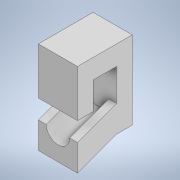
# Autodesk Inventor part: top_part
Saved by Autodesk Inventor 2021 (Build 250183000, 183)
## iProperties
Created: 2021-04-02
Part Number: top_part
Material: Generic
Document SubType Name: Modeling
Designer: Jawal
Density: 1 g/cm^3
Appearance: Default
Author: Jawal
Autodesk Inventor part; units mm, degrees
ref_plane "YZ Plane" through (0, 0, 0) normal (1, 0, 0) x (0, 1, 0)
ref_plane "XZ Plane" through (0, 0, 0) normal (0, 1, 0) x (-1, 0, 0)
sketch "Sketch1" plane through (0, 0, 0) normal (0, 0, 1) x (1, 0, 0)
  line L0 (-12.5, 12.5) -> (12.5, 12.5)
  line L1 (12.5, 12.5) -> (12.5, -37.5)
  line L2 (12.5, -37.5) -> (-12.5, -37.5)
  line L3 (-12.5, -37.5) -> (-12.5, 12.5)
  point P0 (0, 0)
  dimension "d0" = 25
  dimension "d1" = 50
  dimension "d2" = 12.5
  dimension "d3" = 12.5
  constraints: 8 end point, 2 parallel, 1 horizontal, 1 perpendicular
  measures "d0" distance of L0.start L0.end
  measures "d1" distance of L0.end L1.end
  measures "d2" distance from line of L1 point (0, 0)
  measures "d3" distance from line of point (0, 0) L0
extrude "Extrusion1" add sketch "Sketch1" along normal blind 10
sketch "Sketch2" plane through (0, 0, 0) normal (0, 0, -1) x (-1, 0, 0)
  circle A0 centre (0, -33) radius 1.5
  circle A1 centre (0, 0) radius 7.5
  dimension "d7" = 3
  dimension "d8" = 33
  dimension "d17" = 15
  constraints: 2 centre point, 1 coincident
  measures "d7" diameter of A0
  measures "d8" distance of A0.centre point (0, 0)
  measures "d17" diameter of A1
extrude "Extrusion2" add sketch "Sketch2" along normal blind 6 contours A0
sketch "Sketch3" plane through (0, 0, 10) normal (0, 0, 1) x (1, 0, 0)
  arc A0 (7.5, 0) -> (-7.5, 0) centre (0, 0) ccw
  line L0 (-7.5, 0) -> (-12.5, 0)
  line L1 (-12.5, 12.5) -> (-12.5, -37.5) projected
  line L2 (-12.5, 0) -> (-12.5, 12.5)
  line L3 (12.5, 12.5) -> (-12.5, 12.5) projected
  line L4 (12.5, 12.5) -> (12.5, 0)
  line L5 (12.5, -37.5) -> (12.5, 12.5) projected
  line L6 (7.5, 0) -> (12.5, 0)
  dimension "d11" = 15
  constraints: 8 end point, 2 point on circle, 2 point on line, 1 centre point, 1 coincident, 1 collinear, 1 horizontal, 1 perpendicular
  measures "d11" diameter of A0
extrude "Extrusion3" add sketch "Sketch3" along normal blind 15
sketch "Sketch4" plane through (0, 0, 25) normal (0, 0, 1) x (1, 0, 0)
  line L0 (-12.5, 12.5) -> (-12.5, 0) projected
  line L1 (-12.5, 12.5) -> (12.5, 12.5)
  line L2 (12.5, 12.5) -> (12.5, -17.5)
  line L3 (12.5, -17.5) -> (-12.5, -17.5)
  line L4 (-12.5, -17.5) -> (-12.5, 12.5)
  point P0 (0, 0)
  dimension "d14" = 25
  dimension "d21" = 30
  constraints: 8 end point, 2 parallel, 1 horizontal, 1 perpendicular
  measures "d14" distance of L2.end L3.end
  measures "d21" distance of L1.end L2.end
extrude "Extrusion4" add sketch "Sketch4" along normal blind 10
sketch "Sketch5" plane through (0, 0, 0) normal (0, 0, -1) x (-1, 0, 0)
  circle A0 centre (0, 0) radius 7.5
  dimension "d18" = 15
  constraints: 1 centre point, 1 coincident
  measures "d18" diameter of A0
extrude "Extrusion5" cut sketch "Sketch5" against normal blind 10
sketch "Sketch6" plane through (0, 0, 10) normal (0, 0, 1) x (1, 0, 0)
  line L0 (-12.5, -20.5) -> (-12.5, -37.5)
  line L1 (-12.5, -37.5) -> (12.5, -37.5) projected
  line L2 (-12.5, -37.5) -> (12.5, -37.5)
  line L3 (12.5, -37.5) -> (12.5, -20.5)
  line L4 (12.5, -37.5) -> (12.5, 0) projected
  arc A0 (-7.5, -20.5) -> (7.5, -20.5) centre (0, -20.5) ccw
  line L5 (-12.5, -20.5) -> (-7.5, -20.5)
  line L6 (7.5, -20.5) -> (12.5, -20.5)
  line L7 (-12.5, 0) -> (-12.5, -37.5) projected
  line L8 (-12.5, -29) -> (12.5, -29)
  point P0 (0, 0)
  dimension "d22" = 15
  dimension "d23" = 17
  dimension "d24" = 17
  constraints: 12 end point, 3 point on line, 2 horizontal, 2 point on circle, 1 centre point, 1 collinear, 1 perpendicular
  measures "d22" diameter of A0
  measures "d23" distance of L1.end L3.end
  measures "d24" distance of L0.start L0.end
ref_plane "Work Plane1" through (0, -37.5, 0) normal (-1, 0, 0) x (0, 0, 1)
sketch "Sketch8" plane through (0, -37.5, 0) normal (-1, 0, 0) x (0, 0, 1)
  line L0 (10, 0) -> (10, 37.5) projected
  line L1 (10, 8.5) -> (35, -0.5993)
  line L2 (10, 8.5) -> (36.6044, 8.5) construction
  line L3 (0, 0) -> (10, 0) projected
  point P0 (0, 37.5)
  dimension "d26" = 20
  dimension "d27" = 8.5
  dimension "d32" = 25
  constraints: 4 end point, 1 equal length, 1 horizontal, 1 point on line
  measures "d26" angle of L1 L2
  measures "d27" distance between parallel lines of L3 L2
  measures "d32" distance from line of L1.end L0
sweep "Sweep1" add profiles "Sketch6" path "Sketch8" path curves L1
thread "Thread1"
equation "\"d2\" = 0.5 * d0"
equation "\"d24\" = d23"
body "Solid1"
